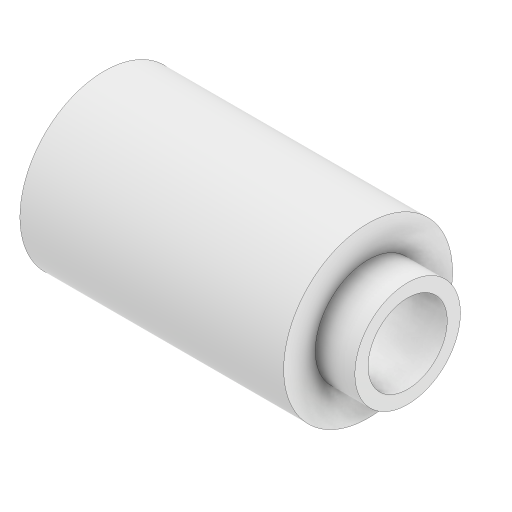
# Autodesk Inventor part: Part1
Saved by Autodesk Inventor 2024.2 (Build 282272000, 272)
## iProperties
Created: 2019-06-28
Part Number: Part1
Material: ポリスチレン
Document SubType Name: Modeling
Designer: Nakamura
Density: 1.021 g/cm^3
Appearance: 滑らか - 白
Mass: 4.80789 g
Surface Area: 35.0593 cm^2
Volume: 4.709 cm^3
Author: Nakamura
Autodesk Inventor part; units mm, degrees
ref_plane "YZ Plane" through (0, 0, 0) normal (1, 0, 0) x (0, 1, 0)
ref_plane "XZ Plane" through (0, 0, 0) normal (0, 1, 0) x (-1, 0, 0)
ref_plane "XY Plane" through (0, 0, 0) normal (0, 0, 1) x (1, 0, 0)
sketch "スケッチ1" plane through (0, 0, 0) normal (0, 0, 1) x (1, 0, 0)
  line L0 (-10, 6.4) -> (10, 6.4)
  line L1 (10, 6.4) -> (10, 3)
  line L2 (10, 3) -> (-10, 3)
  line L3 (0, 0) -> (14.8811, 0)
  line L4 (-10, 6.4) -> (-10, 3)
  point P0 (0, 3)
  dimension "d14" = 6
  dimension "d15" = 12.8
  dimension "d17" = 20
  constraints: 11 end point, 2 vertical, 1 horizontal, 1 midpoint, 1 vertical alignment
  measures "d14" diameter of L2 L3
  measures "d15" diameter of L0 L3
  measures "d17" distance of L0.start L0.end
revolve "回転1" add sketch "スケッチ1" angle 360 about axis through (0, 0, 0) along (1, 0, 0)
sketch "Sketch3" plane through (10, 0, 0) normal (1, 0, 0) x (0, 0, -1)
  circle A0 centre (0, 0) radius 3 projected
  circle A1 centre (0, 0) radius 4
  dimension "d18" = 8
  constraints: 1 centre point, 1 coincident
  measures "d18" diameter of A1
extrude "Extrusion1" add sketch "Sketch3" along normal blind 3
